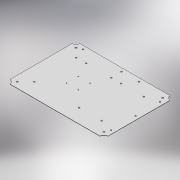
# Autodesk Inventor part: MetalSheet
Saved by Autodesk Inventor 2020 (Build 240168000, 168)
## iProperties
Created: 2020-07-09
Part Number: MetalSheet
Material: Generic
Document SubType Name: Sheet Metal
Designer: nicoc
Density: 1 g/cm^3
Sheet Metal Rule: Default_mm
Appearance: Default
Mass: 86.4316 g
Surface Area: 1743.83 cm^2
Volume: 86.4316 cm^3
Author: nicoc
Autodesk Inventor part; units mm, degrees
ref_plane "YZ Plane" through (0, 0, 0) normal (1, 0, 0) x (0, 1, 0)
ref_plane "XZ Plane" through (0, 0, 0) normal (0, 1, 0) x (-1, 0, 0)
ref_plane "XY Plane" through (0, 0, 0) normal (0, 0, 1) x (1, 0, 0)
sketch "Sketch1" plane through (0, 0, 0) normal (0, 1, 0) x (-1, 0, 0)
  line L0 (0, 0) -> (350, 0)
  line L1 (350, 0) -> (350, -250)
  line L2 (350, -250) -> (0, -250)
  line L3 (0, -250) -> (0, 0)
  dimension "d0" = 250
  dimension "d1" = 350
  constraints: 8 end point, 2 parallel, 1 horizontal, 1 perpendicular
  measures "d0" distance of L2.end L0.start
  measures "d1" distance of L1.end L2.end
extrude "Extrusion1" add sketch "Sketch1" along normal blind 1
sketch "Sketch2" plane through (0, 1, 0) normal (0, 1, 0) x (1, 0, 0)
  line L0 (-350, 0) -> (0, 0) projected
  line L1 (0, 0) -> (0, 250) projected
  line L2 (0, 250) -> (-350, 250) projected
  line L3 (-350, 250) -> (-350, 0) projected
  circle A0 centre (2, -2) radius 16.5
  circle A1 centre (-352, -2) radius 16.5
  circle A2 centre (-352, 252) radius 16.5
  circle A3 centre (2, 252) radius 16.5
  dimension "d9" = 2
  dimension "d10" = 2
  dimension "d11" = 33
  dimension "d12" = 2
  dimension "d13" = 2
  dimension "d14" = 33
  dimension "d15" = 2
  dimension "d16" = 2
  dimension "d17" = 33
  dimension "d18" = 2
  dimension "d19" = 2
  dimension "d20" = 33
  constraints: 4 centre point, 4 coincident
  measures "d9" distance from line of point (2, -2) L1
  measures "d10" distance from line of L0 point (2, -2)
  measures "d11" diameter of A0
  measures "d12" distance from line of point (-352, -2) L3
  measures "d13" distance from line of point (-352, -2) L0
  measures "d14" diameter of A1
  measures "d15" distance from line of point (-352, 252) L2
  measures "d16" distance from line of A2.centre L3
  measures "d17" diameter of A2
  measures "d18" distance from line of A3.centre L2
  measures "d19" distance from line of L1 A3.centre
  measures "d20" diameter of A3
extrude "Extrusion2" cut sketch "Sketch2" against normal blind 1 contours L3 A1 L0 | L0 A1 L3 | A0 L1 L0 | L0 L1 A0 | A2 L2 L3 | L3 L2 A2 | A3 L2 L1 | L1 L2 A3
sketch "Sketch3" plane through (0, 1, 0) normal (0, 1, 0) x (1, 0, 0)
  line L0 (-335.6217, 0) -> (-14.3783, 0) projected
  line L1 (0, 14.3783) -> (0, 235.6217) projected
  line L2 (-14.3783, 250) -> (-335.6217, 250) projected
  line L3 (-350, 235.6217) -> (-350, 14.3783) projected
  point P0 (0, 0)
  point P1 (-20, 20)
  point P2 (-20, 230)
  point P3 (-330, 230)
  point P4 (-330, 20)
  dimension "d23" = 20
  dimension "d24" = 20
  dimension "d25" = 20
  dimension "d26" = 20
  dimension "d27" = 20
  dimension "d28" = 20
  dimension "d29" = 20
  dimension "d30" = 20
  measures "d23" distance from line of point (-20, 20) L0
  measures "d24" distance from line of point (-20, 20) L1
  measures "d25" distance from line of point (-20, 230) L1
  measures "d26" distance from line of L2 point (-20, 230)
  measures "d27" distance from line of L2 point (-330, 230)
  measures "d28" distance from line of L3 point (-330, 230)
  measures "d29" distance from line of L3 point (-330, 20)
  measures "d30" distance from line of L0 point (-330, 20)
hole "Hole1" at (-20, 1, -20) at (-20, 1, -230) at (-330, 1, -230) at (-330, 1, -20) direction (0, -1, 0) diameter 6.4 end through all
sketch "Sketch5" plane through (0, 1, 0) normal (0, 1, 0) x (1, 0, 0)
  line L0 (0, 14.3783) -> (0, 235.6217) projected
  line L1 (-14.3783, 250) -> (-335.6217, 250) projected
  line L2 (-335.6217, 0) -> (-14.3783, 0) projected
  line L3 (-350, 235.6217) -> (-350, 14.3783) projected
  point P0 (0, 0)
  point P1 (-12.5, 37.5)
  point P2 (-12.5, 125)
  point P3 (-12.5, 212.5)
  point P4 (-112.5, 237.5)
  point P5 (-175, 237.5)
  point P6 (-312.5, 237.5)
  dimension "d38" = 12.5
  dimension "d39" = 12.5
  dimension "d40" = 12.5
  dimension "d41" = 37.5
  dimension "d42" = 37.5
  dimension "d43" = 125
  dimension "d44" = 112.5
  dimension "d45" = 175
  dimension "d46" = 37.5
  dimension "d47" = 12.5
  dimension "d48" = 12.5
  dimension "d49" = 12.5
  measures "d38" distance from line of point (-12.5, 212.5) L0
  measures "d39" distance from line of point (-12.5, 125) L0
  measures "d40" distance from line of L0 point (-12.5, 37.5)
  measures "d41" distance from line of point (-12.5, 212.5) L1
  measures "d42" distance from line of point (-12.5, 37.5) L2
  measures "d43" distance from line of point (-12.5, 125) L2
  measures "d44" distance from line of point (-112.5, 237.5) L0
  measures "d45" distance from line of point (-175, 237.5) L0
  measures "d46" distance from line of point (-312.5, 237.5) L3
  measures "d47" distance from line of point (-312.5, 237.5) L1
  measures "d48" distance from line of L1 point (-175, 237.5)
  measures "d49" distance from line of L1 point (-112.5, 237.5)
hole "Hole2" at (-12.5, 1, -37.5) at (-12.5, 1, -125) at (-12.5, 1, -212.5) at (-112.5, 1, -237.5) at (-175, 1, -237.5) at (-312.5, 1, -237.5) direction (0, -1, 0) diameter 5.3 end through all
sketch "Sketch6" plane through (0, 1, 0) normal (0, 1, 0) x (1, 0, 0)
  line L0 (0, 14.3783) -> (0, 235.6217) projected
  line L1 (-335.6217, 0) -> (-14.3783, 0) projected
  line L2 (-14.3783, 250) -> (-335.6217, 250) projected
  point P0 (0, 0)
  point P1 (-58, 50)
  point P2 (-58, 200)
  dimension "d57" = 58
  dimension "d58" = 50
  dimension "d59" = 50
  dimension "d60" = 58
  measures "d57" distance from line of point (-58, 50) L0
  measures "d58" distance from line of L1 point (-58, 50)
  measures "d59" distance from line of L2 point (-58, 200)
  measures "d60" distance from line of L0 point (-58, 200)
hole "Hole3" at (-58, 1, -50) at (-58, 1, -200) direction (0, -1, 0) diameter 5.3 end through all
sketch "Sketch7" plane through (0, 1, 0) normal (0, 1, 0) x (1, 0, 0)
  line L0 (0, 14.3783) -> (0, 235.6217) projected
  line L1 (-335.6217, 0) -> (-14.3783, 0) projected
  line L2 (-14.3783, 250) -> (-335.6217, 250) projected
  point P0 (0, 0)
  point P1 (-139, 50)
  point P2 (-139, 200)
  point P3 (-174, 200)
  point P4 (-264, 200)
  point P5 (-299, 50)
  point P6 (-299, 200)
  dimension "d68" = 139
  dimension "d69" = 139
  dimension "d70" = 50
  dimension "d71" = 50
  dimension "d79" = 50
  dimension "d80" = 50
  dimension "d81" = 50
  dimension "d82" = 50
  dimension "d83" = 90
  dimension "d84" = 35
  dimension "d85" = 160
  dimension "d86" = 160
  measures "d68" distance from line of point (-139, 50) L0
  measures "d69" distance from line of L0 point (-139, 200)
  measures "d70" distance from line of point (-139, 50) L1
  measures "d71" distance from line of L2 point (-139, 200)
  measures "d79" distance from line of L2 point (-174, 200)
  measures "d80" distance from line of L2 point (-264, 200)
  measures "d81" distance from line of L1 point (-299, 50)
  measures "d82" distance from line of L2 point (-299, 200)
  measures "d83" distance of point (-264, 200) point (-174, 200)
  measures "d84" distance of point (-174, 200) point (-139, 200)
  measures "d85" distance of point (-299, 200) point (-139, 200)
  measures "d86" horizontal distance of point (-299, 50) point (-139, 200)
hole "Hole4" at (-139, 1, -50) at (-139, 1, -200) at (-174, 1, -200) at (-264, 1, -200) at (-299, 1, -50) at (-299, 1, -200) direction (0, -1, 0) diameter 5.3 end through all
sketch "Sketch8" plane through (0, 1, 0) normal (0, 1, 0) x (1, 0, 0)
  line L0 (0, 14.3783) -> (0, 235.6217) projected
  line L1 (-335.6217, 0) -> (-14.3783, 0) projected
  point P0 (0, 0)
  point P1 (-237.5, 104)
  point P2 (-237.5, 146)
  point P3 (-195.5, 104)
  point P4 (-195.5, 146)
  dimension "d87" = 42
  dimension "d88" = 42
  dimension "d89" = 42
  dimension "d90" = 195.5
  dimension "d91" = 195.5
  dimension "d92" = 42
  dimension "d93" = 104
  dimension "d94" = 104
  measures "d87" distance of point (-195.5, 146) point (-195.5, 104)
  measures "d88" distance of point (-237.5, 146) point (-237.5, 104)
  measures "d89" distance of point (-237.5, 146) point (-195.5, 146)
  measures "d90" distance from line of point (-195.5, 104) L0
  measures "d91" distance from line of L0 point (-195.5, 146)
  measures "d92" distance of point (-195.5, 104) point (-237.5, 104)
  measures "d93" distance from line of L1 point (-195.5, 104)
  measures "d94" distance from line of L1 point (-237.5, 104)
hole "Hole5" at (-237.5, 1, -104) at (-237.5, 1, -146) at (-195.5, 1, -104) at (-195.5, 1, -146) direction (0, -1, 0) diameter 2.7 end through all
equation "\"d14\" = d11"
equation "\"d17\" = d11"
equation "\"d20\" = d11"
equation "\"d25\" = d24"
equation "\"d26\" = d23"
equation "\"d27\" = d23"
equation "\"d28\" = d24"
equation "\"d29\" = d24"
equation "\"d30\" = d23"
equation "\"d36\" = Thickness"
equation "\"d39\" = d38"
equation "\"d40\" = d38"
equation "\"d42\" = d41"
equation "\"d48\" = d47"
equation "\"d49\" = d47"
equation "\"d55\" = Thickness"
equation "\"d59\" = d58"
equation "\"d60\" = d57"
equation "\"d66\" = Thickness"
equation "\"d69\" = d68"
equation "\"d71\" = d70"
equation "\"d80\" = d79"
equation "\"d81\" = d70"
equation "\"d82\" = d70"
equation "\"d86\" = d85"
equation "\"d77\" = Thickness"
equation "\"d88\" = d87"
equation "\"d91\" = d90"
equation "\"d92\" = d89"
equation "\"d94\" = d93"
equation "\"d100\" = Thickness"
equation "\"BendRadius\" = Thickness"
equation "\"BendReliefWidth\" = Thickness"
equation "\"BendReliefDepth\" = 0.5 * Thickness"
equation "\"CornerReliefSize\" = 4 * Thickness"
equation "\"MinimumRemnant\" = 2 * Thickness"
equation "\"TransitionRadius\" = BendRadius"
equation "\"JacobiRadiusSize\" = BendRadius"
equation "\"GapSize\" = Thickness"
equation "\"Thickness\" = 0.5"
body "Solid1"
